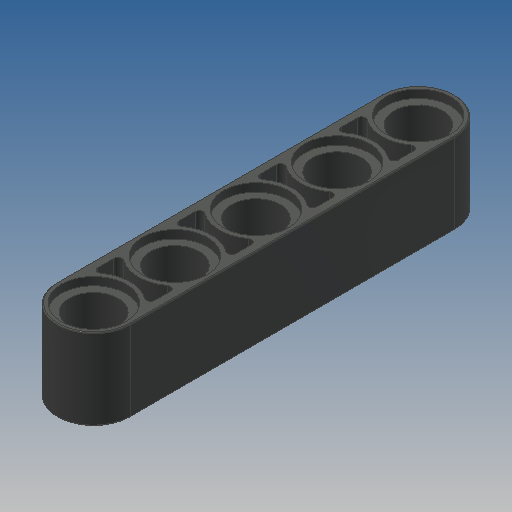
# Autodesk Inventor part: 32316-DkBluishGray
Saved by Autodesk Inventor 2022.2 (Build 262287000, 287)
## iProperties
Created: 2012-03-21
Part Number: 32316-DkBluishGray
Document SubType Name: Modeling
Designer: D. Kohfeld
Density: 1.06 g/cm^3
Material: ABS Plastic
Mass: 1.20936 g
Surface Area: 20.8219 cm^2
Volume: 1.14091 cm^3
Appearance: DkBluishGray
Author: D. Kohfeld
Autodesk Inventor part; units mm, degrees
ref_plane "YZ Plane" through (0, 0, 0) normal (1, 0, 0) x (0, 1, 0)
ref_plane "XZ Plane" through (0, 0, 0) normal (0, 1, 0) x (-1, 0, 0)
ref_plane "XY Plane" through (0, 0, 0) normal (0, 0, 1) x (1, 0, 0)
sketch "Sketch1" plane through (0, 0, 0) normal (0, 0, 1) x (1, 0, 0)
  line L0 (3.6, -16) -> (3.6, 16)
  line L1 (-3.6, 16) -> (-3.6, -16)
  arc A0 (3.6, 16) -> (-3.6, 16) centre (0, 16) ccw
  circle A1 centre (0, 8) radius 2.4
  circle A2 centre (0, 8) radius 3.2
  circle A3 centre (0, 0) radius 3.2
  circle A4 centre (0, 0) radius 2.4
  line L2 (0, 0) -> (0, 8) construction
  line L3 (-2.8, 5.7373) -> (-2.8, 2.2627)
  line L4 (2.8, 5.7373) -> (2.8, 2.2627)
  arc A5 (-2.8, 5.7373) -> (2.8, 5.7373) centre (0, 8) ccw
  arc A6 (2.8, 2.2627) -> (-2.8, 2.2627) centre (0, 0) ccw
  arc A7 (-3.6, -16) -> (3.6, -16) centre (0, -16) ccw
  circle A8 centre (0, -8) radius 3.2
  circle A9 centre (0, -8) radius 2.4
  line L5 (0, 0) -> (0, -8) construction
  line L6 (-2.8, -2.2627) -> (-2.8, -5.7373)
  line L7 (2.8, -2.2627) -> (2.8, -5.7373)
  arc A10 (-2.8, -2.2627) -> (2.8, -2.2627) centre (0, 0) ccw
  arc A11 (2.8, -5.7373) -> (-2.8, -5.7373) centre (0, -8) ccw
  circle A12 centre (0, 16) radius 3.2
  circle A13 centre (0, 16) radius 2.4
  circle A14 centre (0, -16) radius 3.2
  circle A15 centre (0, -16) radius 2.4
  line L8 (0, 16) -> (0, 8) construction
  line L9 (0, -8) -> (0, -16) construction
  line L10 (2.8, 13.7373) -> (2.8, 10.2627)
  line L11 (-2.8, 13.7373) -> (-2.8, 10.2627)
  arc A16 (-2.8, 13.7373) -> (2.8, 13.7373) centre (0, 16) ccw
  arc A17 (2.8, 10.2627) -> (-2.8, 10.2627) centre (0, 8) ccw
  arc A18 (-2.8, -10.2627) -> (2.8, -10.2627) centre (0, -8) ccw
  arc A19 (2.8, -13.7373) -> (-2.8, -13.7373) centre (0, -16) ccw
  line L12 (2.8, -13.7373) -> (2.8, -10.2627)
  line L13 (-2.8, -10.2627) -> (-2.8, -13.7373)
  dimension "d8" = 4.8
  dimension "d9" = 6.4
  dimension "d32" = 7.2
  dimension "d34" = 8
  dimension "d36" = 0.8
  constraints: 28 end point, 20 centre point, 20 point on circle, 16 coincident, 16 equal radius, 10 equal length, 10 parallel, 4 tangent, 2 vertical, 1 collinear
  measures "d8" diameter of A1
  measures "d9" diameter of A2
  measures "d32" diameter of A0
  measures "d34" distance of L2.start L2.end
  measures "d36" distance between parallel lines of L1 L3
extrude "Extrusion1" add sketch "Sketch1" along normal mid plane 8 contours A7 L1 A0 L0 | A2 | A3 | A5 L4 A6 L3 | A8 | A10 L7 A11 L6 | A12 | A14 | L10 A17 L11 A16 | A18 L12 A19 L13
sketch "Sketch6" plane through (0, 0, 4) normal (0, 0, 1) x (1, 0, 0)
  circle A0 centre (0, 0) radius 2.4 projected
  circle A1 centre (0, 8) radius 2.4 projected
  circle A2 centre (0, 0) radius 3.2 projected
  circle A3 centre (0, 8) radius 3.2 projected
  arc A4 (2.8, 2.2627) -> (-2.8, 2.2627) centre (0, 0) ccw projected
  line L0 (-2.8, 5.7373) -> (-2.8, 2.2627) projected
  arc A5 (-2.8, 5.7373) -> (2.8, 5.7373) centre (0, 8) ccw projected
  line L1 (2.8, 5.7373) -> (2.8, 2.2627) projected
  line L2 (-2.8, -2.2627) -> (-2.8, -5.7373) projected
  arc A6 (-2.8, -2.2627) -> (2.8, -2.2627) centre (0, 0) ccw projected
  arc A7 (2.8, -5.7373) -> (-2.8, -5.7373) centre (0, -8) ccw projected
  line L3 (2.8, -2.2627) -> (2.8, -5.7373) projected
  circle A8 centre (0, -8) radius 3.2 projected
  circle A9 centre (0, -8) radius 2.4 projected
  circle A10 centre (0, -16) radius 2.4 projected
  circle A11 centre (0, 16) radius 2.4 projected
  line L4 (2.8, -13.7373) -> (2.8, -10.2627) projected
  arc A12 (2.8, -13.7373) -> (-2.8, -13.7373) centre (0, -16) ccw projected
  arc A13 (-2.8, -10.2627) -> (2.8, -10.2627) centre (0, -8) ccw projected
  line L5 (-2.8, -10.2627) -> (-2.8, -13.7373) projected
  circle A14 centre (0, -16) radius 3.2 projected
  circle A15 centre (0, 16) radius 3.2 projected
  line L6 (2.8, 13.7373) -> (2.8, 10.2627) projected
  arc A16 (-2.8, 13.7373) -> (2.8, 13.7373) centre (0, 16) ccw projected
  arc A17 (2.8, 10.2627) -> (-2.8, 10.2627) centre (0, 8) ccw projected
  line L7 (-2.8, 13.7373) -> (-2.8, 10.2627) projected
extrude "Extrusion7" cut sketch "Sketch6" against normal blind 0.8 contours A2 | A3 | A8 | A14 | A15
extrude "Extrusion8" cut sketch "Sketch6" against normal blind 3.1 contours A4 L0 A5 L1 | A6 L3 A7 L2 | A12 L5 A13 L4 | L6 A17 L7 A16
mirror "Mirror1" about plane through (0, 0, 0) normal (0, 0, 1) of "Extrusion7", "Extrusion8"
fillet "Fillet1" radius 0.4 32 edges at (-2.8, 2.2627, 2.45) (-2.8, 5.7373, 2.45) (2.8, 2.2627, 2.45) (2.8, 5.7373, 2.45) (2.8, 5.7373, -2.45) (2.8, 2.2627, -2.45) (-2.8, 2.2627, -2.45) (-2.8, 5.7373, -2.45) (-2.8, -2.2627, 2.45) (-2.8, -5.7373, 2.45) (2.8, -5.7373, 2.45) (2.8, -2.2627, 2.45) (2.8, -2.2627, -2.45) (2.8, -5.7373, -2.45) (-2.8, -5.7373, -2.45) (-2.8, -2.2627, -2.45) (-2.8, -13.7373, 2.45) (-2.8, -13.7373, -2.45) (-2.8, -10.2627, 2.45) (-2.8, -10.2627, -2.45) (2.8, -13.7373, 2.45) (2.8, -10.2627, 2.45) (2.8, -13.7373, -2.45) (2.8, -10.2627, -2.45) (-2.8, 10.2627, 2.45) (-2.8, 13.7373, 2.45) (-2.8, 10.2627, -2.45) (-2.8, 13.7373, -2.45) (2.8, 10.2627, 2.45) (2.8, 13.7373, 2.45) (2.8, 10.2627, -2.45) (2.8, 13.7373, -2.45)
fillet "Fillet1" radius 0.1 8 edges at (0, -19.6, 4) (-3.6, 0, 4) (0, 19.6, 4) (3.6, 0, 4) (0, 19.6, -4) (-3.6, 0, -4) (0, -19.6, -4) (3.6, 0, -4)
equation "\"lf\" = 0.1"
equation "\"tf\" = 0.4"
body "Solid1"
